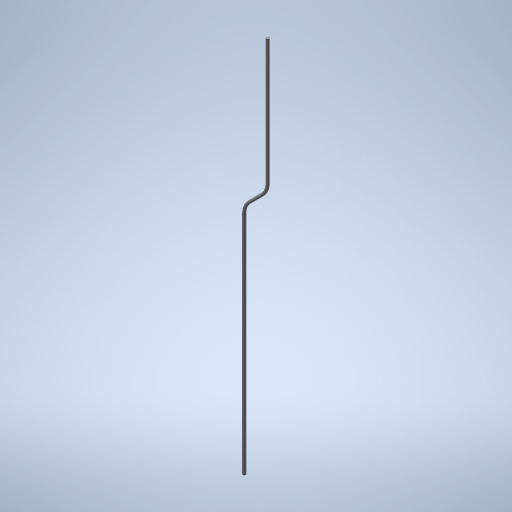
# Autodesk Inventor part: cable meñique
Saved by Autodesk Inventor 2023 (Build 270158000, 158)
## iProperties
Created: 2022-10-18
Part Number: cable meñique
Material: Generic
Document SubType Name: Modeling
Designer: Xiaba
Density: 1 g/cm^3
Appearance: Default
Author: Xiaba
Autodesk Inventor part; units mm, degrees
ref_plane "YZ Plane" through (0, 0, 0) normal (1, 0, 0) x (0, 1, 0)
ref_plane "XZ Plane" through (0, 0, 0) normal (0, 1, 0) x (-1, 0, 0)
ref_plane "XY Plane" through (0, 0, 0) normal (0, 0, 1) x (1, 0, 0)
sketch "Sketch1" plane through (0, 0, 0) normal (0, 1, 0) x (-1, 0, 0)
  circle A0 centre (0, 0) radius 0.45
  dimension "d0" = 0.9
  constraints: 1 centre point, 1 coincident
  measures "d0" diameter of A0
sketch "Sketch2" plane through (0, 0, 0) normal (0, 0, 1) x (1, 0, 0)
  line L0 (0, 0) -> (0, 0.1)
  line L1 (0, 0.1) -> (0, 68.0289)
  line L2 (1.4645, 71.5645) -> (5.6066, 75.7066)
  line L3 (7.0711, 79.2421) -> (7.0711, 117.1711)
  arc A0 (5.6066, 75.7066) -> (7.0711, 79.2421) centre (2.0711, 79.2421) ccw
  arc A1 (1.4645, 71.5645) -> (0, 68.0289) centre (5, 68.0289) ccw
  point P0 (0, 70.1)
  point P1 (7.0711, 77.1711)
  dimension "d1" = 0.1
  dimension "d6" = 10
  dimension "d7" = 40
  dimension "d8" = 5
  dimension "d9" = 5
  constraints: 8 end point, 4 point on circle, 4 point on line, 4 tangent, 3 vertical, 2 centre point
  measures "d1" distance of L0.start L0.end
  measures "d6" distance of point (0, 70.1) point (7.071, 77.171)
  measures "d7" distance of point (7.071, 77.171) L3.end
  measures "d8" radius of A0
  measures "d9" radius of A1
sweep "Sweep2" add profiles "Sketch1" path "Sketch2"
body "Solid2"
